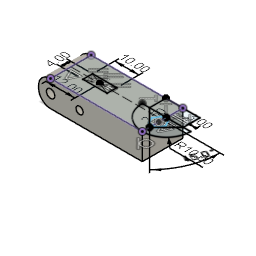
_penhoude.71a9cce0-3994-4f7b-b995-d0deb1614a8e (Autodesk Fusion 360 design; units mm, degrees)
Autodesk Fusion 360 part; units mm, degrees
sketch "Sketch1" plane through (0, 0, 0) normal (0, 0, 1) x (1, 0, 0)
  line L0 (-5, -5.4) -> (38, -5.4)
  line L1 (-5, 5.4) -> (-5, -5.4)
  line L2 (38, -5.4) -> (38, 5.4)
  line L3 (38, 5.4) -> (-5, 5.4)
  circle A0 centre (0, 0) radius 1.75
  circle A1 centre (12, 0) radius 1.5
  line L4 (-5, -5.4) -> (38, 5.4) construction
  line L5 (38, -5.4) -> (-5, 5.4) construction
  line L6 (-5, 0) -> (38, 0) construction
  dimension "d1" = 3.5
  dimension "d2" = 3
  dimension "d3" = 10.8
  dimension "d4" = 43
  dimension "d5" = 5
  dimension "d6" = 17
  constraint midpoint L1 L6.start
  constraint midpoint L2 L6.end
  constraint coincident A0.centre L6
  constraint coincident A1.centre L6
  constraint coincident A0.centre origin
  constraint perpendicular L1 L3
  constraint perpendicular L0 L1
  constraint perpendicular L2 L3
  constraint horizontal L3
  measures "d1" diameter of A0
  measures "d2" diameter of A1
  measures "d3" distance of L0.end L2.end
  measures "d4" distance of L1.start L2.end
  measures "d5" distance of A0.centre L1
  measures "d6" distance of L1 A1.centre
extrude "Extrude1" add sketch "Sketch1" along normal blind 16.8
fillet "Fillet1" radius 5 2 edges at (-5, 5.4, 8.4) (-5, -5.4, 8.4)
sketch "Sketch2" plane through (0, 5.4, 0) normal (0, 1, 0) x (-1, 0, 0)
  line L0 (0, 16.8) -> (-38, 16.8)
  line L1 (-38, 16.8) -> (-38, 0)
  line L2 (-38, 0) -> (0, 0)
  line L3 (0, 8.4) -> (-38, 8.4) construction
  line L4 (-17, 10.4) -> (-7, 10.4)
  line L5 (-7, 10.4) -> (-7, 6.4)
  line L6 (-7, 6.4) -> (-17, 6.4)
  line L7 (-17, 6.4) -> (-17, 10.4)
  line L8 (-17, 10.4) -> (-7, 6.4) construction
  line L9 (-7, 10.4) -> (-17, 6.4) construction
  line L10 (-28, 6.8) -> (-48, 6.8)
  line L11 (-31, 6.8) -> (-38, 13.8)
  line L12 (-38, 13.8) -> (-45, 6.8)
  arc A0 (-28, 6.8) -> (-48, 6.8) centre (-38, 6.8) ccw
  line L13 (-31, 6.8) -> (-31, 0)
  line L14 (-45, 0) -> (-45, 6.8)
  line L15 (-45, 0) -> (-31, 0)
  line L16 (0, 0) -> (0, 16.8)
  line L17 (-36.5376, 7.5111) -> (-35.1133, 10.022)
  line L18 (-35.1133, 10.022) -> (-36.5757, 12.5109)
  line L19 (-36.5757, 12.5109) -> (-39.4624, 12.4889)
  line L20 (-39.4624, 12.4889) -> (-40.8867, 9.978)
  line L21 (-40.8867, 9.978) -> (-39.4243, 7.4891)
  line L22 (-39.4243, 7.4891) -> (-36.5376, 7.5111)
  point P0 (-12, 8.4)
  point P1 (-38, 10)
  dimension "d11" = 10
  dimension "d12" = 4
  dimension "d17" = 45
  dimension "d60" = 3
  dimension "d61" = 10
  dimension "d73" = 12
  dimension "d74" = 2.5
  constraint horizontal L4
  constraint perpendicular L4 L5
  constraint parallel L4 L6
  constraint parallel L5 L7
  constraint coincident L8 P0
  constraint coincident L9 P0
  constraint coincident L3 P0
  constraint coincident L10 L11.start
  constraint perpendicular L11 L12
  constraint midpoint L10 A0.centre
  constraint tangent L0 A0
  constraint coincident L10 L12.end
  constraint midpoint L1 L3.end
  constraint horizontal L10
  constraint coincident A0.start L10
  constraint coincident L2 L13.end
  constraint perpendicular L2 L13
  constraint perpendicular L13 L15
  constraint perpendicular L14 L15
  constraint midpoint L3.start L16
  constraint coincident L1 A0.centre
  constraint coincident L1 L11.end
  constraint coincident L1 P1
  measures "d11" distance of L5.end L6.end
  measures "d12" distance of L4.end L5.end
  measures "d17" angle of L3 L11
  measures "d60" distance of L10.end L12.end
  measures "d61" radius of A0
  measures "d73" distance of P0 L16
  measures "d74" distance of P1 L22
extrude "Extrude2" [rolled back] taper angle 10
sketch "Sketch3" plane through (0, 5.4, 0) normal (0, 1, 0) x (-1, 0, 0)
  line L0 (-12, 8) -> (11.0868, 8) construction
  line L1 (0, 16.8) -> (-9.1776, 10.0698)
  line L2 (0, 16.8) -> (-38, 16.8)
  circle A0 centre (-28.273, 16.8) radius 0.75
  line L3 (-15.3823, 8.9) -> (-49, 8.9)
  line L4 (0, 8.4) -> (-38, 8.4)
  line L5 (-21, 8.9) -> (-13.0265, 11.3461)
  circle A1 centre (-12, 8) radius 3.5
  line L6 (-17, 10.4) -> (-7, 10.4)
  line L7 (0, 16.8) -> (-38, 16.8)
  line L8 (-38, 8.9) -> (-38, 16.8)
  line L9 (-17, 6.4) -> (-17, 10.4)
  line L10 (-7, 6.4) -> (-17, 6.4)
  line L11 (-7, 10.4) -> (-7, 6.4)
  line L12 (-17, 10.4) -> (-7, 10.4)
  line L13 (0, 16.8) -> (5, 16.8)
  line L14 (5, 16.8) -> (5, 0)
  line L15 (5, 0) -> (0, 0)
  line L16 (0, 0) -> (-38, 0)
  line L17 (-38, 0) -> (-38, 16.8)
  line L18 (0, 16.8) -> (-38, 16.8)
  line L19 (0, 0) -> (0, 16.8)
  point P0 (-12, 8.4)
  point P1 (-28.273, 16.8)
  point P2 (-12, 8)
  point P3 (-12, 8)
  point P4 (-12, 8)
  point P5 (-12, 8)
  point P6 (-12, 8)
  dimension "d25" = 1.5
  dimension "d27" = 9
  dimension "d28" = 7
  dimension "d29" = 18.5
  dimension "d58" = 0.5
  constraint horizontal L0
  constraint coincident L1.start L2
  constraint coincident P1 A0.centre
  constraint parallel L3 L4
  constraint coincident L3 L5.start
  constraint tangent L5 A1
  constraint coincident L3.start A1
  constraint coincident L5.end A1
  constraint coincident P6 P5
  constraint coincident L1 P6
  constraint coincident L1.end A1
  constraint coincident L2 P1
  constraint coincident L1.start L2.start
  constraint coincident L3 L8.start
  constraint coincident L2.end L7.end
  constraint perpendicular L2 L8
  constraint coincident L2.end L8
  constraint collinear L2 L7
  constraint coincident L1.start L19
  measures "d25" diameter of A0
  measures "d27" horizontal distance of L5.start P6
  measures "d28" diameter of A1
  measures "d29" distance of P1 P6
  measures "d58" distance of L3 L4
extrude "Extrude3" [rolled back] along distance 11 taper angle 0
extrude "Extrude4" [rolled back] along distance 2 taper angle 0
extrude "Extrude5" [rolled back] profile offset 0 along distance 17 taper angle 0 against distance 10 side2taper angle 0
extrude "Extrude6" [rolled back] taper angle 0 side2taper angle 0
sketch "Sketch4" plane through (31, 0, 0) normal (1, 0, 0) x (0, 0, -1)
  line L0 (-6.8, -5.4) -> (0, -5.4)
  line L1 (0, -5.4) -> (0, 5.4)
  line L2 (0, 5.4) -> (-6.8, 5.4)
  line L3 (-6.8, 5.4) -> (-6.8, -5.4)
  line L4 (-16.8, 16.4) -> (-16.8, -5.4)
  line L5 (-16.8, -5.4) -> (-6.8, -5.4)
  line L6 (-6.8, -5.4) -> (0, -5.4)
  line L7 (0, -5.4) -> (0, 5.4)
  line L8 (0, 5.4) -> (-6.8, 5.4)
  line L9 (-6.8, -5.4) -> (-6.8, 5.4)
  line L10 (-13.9414, 22.4) -> (-13.9414, 16.4)
  line L11 (-6.8, 22.4) -> (-13.9414, 22.4)
  line L12 (-6.8, 5.4) -> (-6.8, 22.4)
  line L13 (-6.8, 5.4) -> (-10.8, 9.4)
  line L14 (-10.8, 9.4) -> (-10.8, 13.4)
  line L15 (-10.8, 13.4) -> (-6.8, 17.4)
  line L16 (-6.8, 17.4) -> (-6.8, 5.4)
  dimension "d64" = 45
  dimension "d65" = 45
  dimension "d66" = 12
  dimension "d67" = 4
  constraint coincident L2.end L3.start
  constraint coincident L12 L15.end
  measures "d64" angle of L12 L13
  measures "d65" angle of L12 L15
  measures "d66" distance of L2.end L15.end
  measures "d67" distance of L12 L14
fillet "Fillet3" [rolled back] radius 1.5
extrude "Extrude7" [rolled back] along distance -9 taper angle 0 profile offset 0 against distance -17 side2taper angle 0
